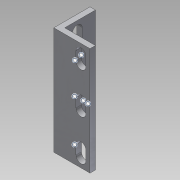
# Autodesk Inventor part: Universal L Bracket
Saved by Autodesk Inventor 2016 (Build 200138000, 138)
## iProperties
Created: 2013-06-26
Part Number: Universal L Bracket
Material: Aluminum 6061
Document SubType Name: Modeling
Designer: Jon Hollander
Density: 2.71 g/cm^3
Mass: 15.4279 g
Surface Area: 48.6592 cm^2
Volume: 5.69295 cm^3
Appearance: Aluminum - Flat
RuleStatus: InUse
Author: Jon Hollander
Autodesk Inventor part; units mm, degrees
ref_plane "YZ Plane" through (0, 0, 0) normal (1, 0, 0) x (0, 1, 0)
ref_plane "XZ Plane" through (0, 0, 0) normal (0, 1, 0) x (-1, 0, 0)
ref_plane "XY Plane" through (0, 0, 0) normal (0, 0, 1) x (1, 0, 0)
sketch "Sketch1" plane through (0, 0, 0) normal (0, 0, 1) x (1, 0, 0)
  line L0 (0, 0) -> (0, 20)
  line L1 (0, 20) -> (3, 20)
  line L2 (3, 20) -> (3, 3)
  line L3 (3, 3) -> (20, 3)
  line L4 (20, 3) -> (20, 0)
  line L5 (20, 0) -> (0, 0)
  dimension "d0" = 20
  dimension "d1" = 3
  dimension "d2" = 17
  dimension "d3" = 17
  constraints: 12 end point, 3 parallel, 2 perpendicular, 1 vertical
  measures "d0" distance of L0.start L0.end
  measures "d1" distance of L0.end L1.end
  measures "d2" distance of L1.end L2.end
  measures "d3" distance of L2.end L3.end
extrude "Extrusion1" add sketch "Sketch1" along normal blind 59.6
sketch "Sketch2" plane through (3, 3, 0) normal (0, 1, 0) x (1, 0, 0)
  line L0 (0, 0) -> (17, 0) projected
  line L1 (17, -59.6) -> (0, -59.6) projected
  line L2 (17, 0) -> (17, -59.6) projected
  line L3 (12, -59.6) -> (12, 0) construction
  line L4 (12, -12.55) -> (12, -12.55)
  line L5 (9.25, -9.8) -> (9.25, -4.8)
  line L6 (12, -2.05) -> (12, -2.05)
  line L7 (14.75, -4.8) -> (14.75, -9.8)
  line L8 (14.75, -12.55) -> (9.25, -2.05) construction
  line L9 (9.25, -12.55) -> (14.75, -2.05) construction
  arc A0 (9.25, -9.8) -> (12, -12.55) centre (12, -9.8) ccw
  arc A1 (12, -12.55) -> (14.75, -9.8) centre (12, -9.8) ccw
  arc A2 (14.75, -4.8) -> (12, -2.05) centre (12, -4.8) ccw
  arc A3 (12, -2.05) -> (9.25, -4.8) centre (12, -4.8) ccw
  point P0 (-3, 0)
  point P1 (12, -7.3)
  dimension "bottom_row_offset" = 5
  dimension "d7" = 5.5
  dimension "hole_length" = 10.5
  dimension "bottom_hole_edge_offset" = 2.05
  dimension "d10" = 2.75
  constraints: 14 end point, 11 point on line, 8 point on circle, 8 tangent, 4 centre point, 3 equal radius, 3 parallel, 2 midpoint, 1 horizontal, 1 perpendicular
  measures "bottom_row_offset" distance between parallel lines of L2 L3
  measures "d7" distance of L8.end L9.end
  measures "hole_length" distance of L9.start L8.end
  measures "bottom_hole_edge_offset" distance between parallel lines of L0 L6
  measures "d10" radius of A0
extrude "Extrusion2" cut sketch "Sketch2" against normal through all
sketch "Sketch3" plane through (3, 3, 0) normal (1, 0, 0) x (0, 0, -1)
  line L0 (0, 17) -> (0, 0) projected
  line L1 (0, 17) -> (-59.6, 17) projected
  line L2 (-59.6, 0) -> (-59.6, 17) projected
  line L3 (-59.6, 7) -> (0, 7) construction
  line L4 (-9.8, 9.75) -> (-4.8, 9.75)
  line L5 (-2.05, 7) -> (-2.05, 7)
  line L6 (-4.8, 4.25) -> (-9.8, 4.25)
  line L7 (-12.55, 7) -> (-12.55, 7)
  line L8 (-12.55, 9.75) -> (-2.05, 4.25) construction
  line L9 (-2.05, 9.75) -> (-12.55, 4.25) construction
  arc A0 (-9.8, 9.75) -> (-12.55, 7) centre (-9.8, 7) ccw
  arc A1 (-12.55, 7) -> (-9.8, 4.25) centre (-9.8, 7) ccw
  arc A2 (-4.8, 4.25) -> (-2.05, 7) centre (-4.8, 7) ccw
  arc A3 (-2.05, 7) -> (-4.8, 9.75) centre (-4.8, 7) ccw
  point P0 (0, -3)
  point P1 (-7.3, 7)
  dimension "top_row_offset" = 10
  dimension "d14" = 10.5
  dimension "d15" = 5.5
  dimension "d16" = 2.75
  dimension "d17" = 2.05
  constraints: 14 end point, 11 point on line, 8 point on circle, 8 tangent, 4 centre point, 3 equal radius, 2 midpoint, 2 parallel, 2 perpendicular, 1 horizontal
  measures "top_row_offset" distance between parallel lines of L1 L3
  measures "d14" distance of L8.end L9.end
  measures "d15" distance of L9.start L8.end
  measures "d16" radius of A0
  measures "d17" distance of L3.end L5.end
extrude "Extrusion3" cut sketch "Sketch3" against normal through all
pattern_linear "Rectangular Pattern1" count 3 spacing 22.5 along (0, 0, 1) of "Extrusion2", "Extrusion3"
equation "\"d14\" = hole_length"
equation "\"d17\" = bottom_hole_edge_offset"
equation "\"hole_number\" = 3"
body "Solid1"
